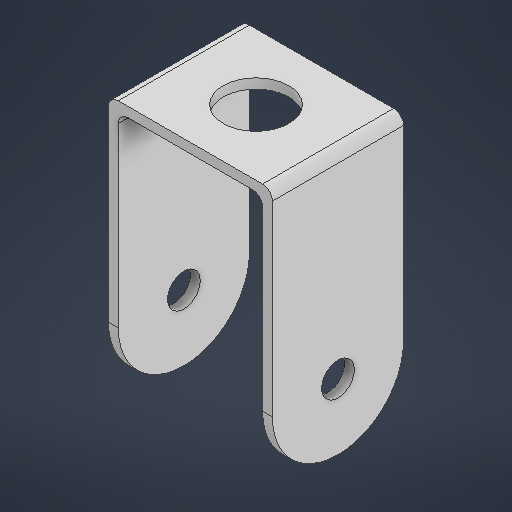
# Autodesk Inventor part: suporte
Saved by Autodesk Inventor 2027 (Build 310192060, 192F)
## iProperties
Created: 2026-08-06
Part Number: suporte
Material: Genérico
Document SubType Name: Modeling
Designer: labsfiap
Density: 1 g/cm^3
Appearance: Padrão
Author: labsfiap
Autodesk Inventor part; units mm, degrees
ref_plane "YZ Plane" through (0, 0, 0) normal (1, 0, 0) x (0, 1, 0)
ref_plane "XZ Plane" through (0, 0, 0) normal (0, 1, 0) x (-1, 0, 0)
ref_plane "XY Plane" through (0, 0, 0) normal (0, 0, 1) x (1, 0, 0)
sketch "Esboço1" plane through (0, 0, 0) normal (0, 0, 1) x (1, 0, 0)
  line L0 (0, 0) -> (0, 80)
  line L1 (0, 80) -> (50, 80)
  line L2 (50, 80) -> (50, 0)
  line L3 (47, 0) -> (47, 77)
  line L4 (47, 77) -> (3, 77)
  line L5 (3, 77) -> (3, 0)
  line L6 (0, 0) -> (3, 0)
  line L7 (47, 0) -> (50, 0)
  dimension "d0" = 80
  dimension "d1" = 3
  dimension "d2" = 3
  dimension "d3" = 50
  dimension "d4" = 3
  constraints: 16 end point, 2 perpendicular, 2 vertical, 1 collinear, 1 horizontal
  measures "d0" distance of L1.end L2.end
  measures "d1" distance between parallel lines of L2 L3
  measures "d2" distance between parallel lines of L5 L0
  measures "d3" distance between parallel lines of L2 L0
  measures "d4" distance between parallel lines of L1 L4
extrude "Extrusão1" add sketch "Esboço1" along normal mid plane 40
fillet "Arredondamento1" radius 20 1 edges at (48.5, 0, 20)
fillet "Arredondamento2" radius 20 1 edges at (48.5, 0, -20)
fillet "Arredondamento3" radius 20 1 edges at (1.5, 0, -20)
fillet "Arredondamento4" radius 20 1 edges at (1.5, 0, 20)
fillet "Arredondamento5" radius 3 1 edges at (50, 80, 0)
fillet "Arredondamento6" radius 3 1 edges at (0, 80, 0)
fillet "Arredondamento7" radius 3 1 edges at (3, 77, 0)
fillet "Arredondamento8" radius 3 1 edges at (47, 77, 0)
sketch "Esboço2" plane through (0, 20, 0) normal (-1, 0, 0) x (0, 0, 1)
  circle A0 centre (0, 0) radius 5
  line L0 (20, 60) -> (-20, 60) projected
  point P0 (0, -20)
  dimension "d15" = 10
  dimension "d16" = 60
  constraints: 1 centre point
  measures "d15" diameter of A0
  measures "d16" distance from line of L0 A0.centre
extrude "Extrusão2" cut sketch "Esboço2" against normal blind 50
sketch "Esboço3" plane through (47, 80, 20) normal (0, 1, 0) x (1, 0, 0)
  line L0 (-44, 25) -> (-44, 15) projected
  line L1 (-44, 20) -> (0, 20)
  line L2 (0, 40) -> (0, 0) projected
  circle A0 centre (-22, 20) radius 10
  point P0 (-47, 20)
  dimension "d19" = 20
  constraints: 3 midpoint, 2 end point, 1 centre point
  measures "d19" diameter of A0
extrude "Extrusão3" cut sketch "Esboço3" against normal blind 50
